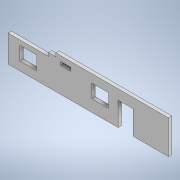
# Autodesk Inventor part: westSideofHouseFacingGarage
Saved by Autodesk Inventor 2020.1 (Build 241239000, 239)
## iProperties
Created: 2019-08-10
Part Number: westSideofHouseFacingGarage
Material: Generic
Document SubType Name: Modeling
Designer: steele
Density: 1 g/cm^3
Appearance: Default
Author: steele
Autodesk Inventor part; units mm, degrees
ref_plane "YZ Plane" through (0, 0, 0) normal (1, 0, 0) x (0, 1, 0)
ref_plane "XZ Plane" through (0, 0, 0) normal (0, 1, 0) x (-1, 0, 0)
ref_plane "XY Plane" through (0, 0, 0) normal (0, 0, 1) x (1, 0, 0)
sketch "Sketch1" plane through (0, 0, 0) normal (0, 0, 1) x (1, 0, 0)
  line L0 (0, 0) -> (3657.6, 0)
  line L1 (3657.6, 0) -> (3657.6, 2438.4)
  line L2 (3657.6, 2438.4) -> (0, 2438.4)
  line L3 (0, 2438.4) -> (0, 0)
  line L4 (3657.6, 0) -> (4318, 0)
  line L5 (4318, 2743.2) -> (3657.6, 2743.2)
  line L6 (3657.6, 2743.2) -> (3657.6, 0)
  line L7 (4318, 0) -> (9956.8, 0)
  line L8 (9956.8, 0) -> (9956.8, 2159)
  line L9 (9956.8, 3048) -> (4318, 3048)
  line L10 (4318, 3048) -> (4318, 0)
  line L11 (9956.8, 0) -> (11328.4, 0)
  line L12 (11328.4, 0) -> (11328.4, 2159)
  line L13 (11328.4, 2159) -> (9956.8, 2159)
  line L14 (9956.8, 2159) -> (9956.8, 0)
  line L15 (9956.8, 0) -> (14528.8, 0)
  line L16 (14528.8, 0) -> (14528.8, 3048)
  line L17 (14528.8, 3048) -> (9956.8, 3048)
  line L18 (9956.8, 3048) -> (9956.8, 0)
  line L19 (4775.2, 2286) -> (5689.6, 2286)
  line L20 (5689.6, 2286) -> (5689.6, 2590.8)
  line L21 (5689.6, 2590.8) -> (4775.2, 2590.8)
  line L22 (4775.2, 2590.8) -> (4775.2, 2286)
  line L23 (4775.2, 2286) -> (5689.6, 2590.8) construction
  line L24 (5689.6, 2286) -> (4775.2, 2590.8) construction
  line L25 (7567.3793, 1088.0908) -> (9091.3793, 1088.0908)
  line L26 (9091.3793, 1088.0908) -> (9091.3793, 2307.2908)
  line L27 (9091.3793, 2307.2908) -> (7567.3793, 2307.2908)
  line L28 (7567.3793, 2307.2908) -> (7567.3793, 1088.0908)
  line L29 (7567.3793, 1088.0908) -> (9091.3793, 2307.2908) construction
  line L30 (9091.3793, 1088.0908) -> (7567.3793, 2307.2908) construction
  line L31 (1066.8, 792.7558) -> (2590.8, 792.7558)
  line L32 (2590.8, 792.7558) -> (2590.8, 2011.9558)
  line L33 (2590.8, 2011.9558) -> (1066.8, 2011.9558)
  line L34 (1066.8, 2011.9558) -> (1066.8, 792.7558)
  line L35 (1066.8, 792.7558) -> (2590.8, 2011.9558) construction
  line L36 (2590.8, 792.7558) -> (1066.8, 2011.9558) construction
  line L37 (4318, 0) -> (4318, 2159)
  line L38 (4318, 2286) -> (4318, 2743.2)
  point P0 (5232.4, 2438.4)
  point P1 (8329.3793, 1697.6908)
  point P2 (1828.8, 1402.3558)
  dimension "d0" = 3657.6
  dimension "d1" = 2438.4
  dimension "d2" = 660.4
  dimension "d3" = 2743.2
  dimension "d4" = 5638.8
  dimension "d5" = 3048
  dimension "d6" = 1371.6
  dimension "d7" = 2159
  dimension "d8" = 4572
  dimension "d9" = 3048
  dimension "d10" = 304.8
  dimension "d11" = 914.4
  dimension "d14" = 1524
  dimension "d15" = 1219.2
  dimension "d16" = 1524
  dimension "d17" = 1219.2
  dimension "d18" = 1828.8
  dimension "d19" = 3200.4
  dimension "d22" = 14528.8
  constraints: 78 end point, 17 parallel, 9 perpendicular, 8 horizontal, 6 midpoint, 2 point on line
  measures "d0" distance of L2.end L1.end
  measures "d1" distance of L1.end L0.end
  measures "d2" distance of L5.end L5.start
  measures "d3" distance of L5.start L4.end
  measures "d4" distance of L9.end L9.start
  measures "d5" distance of L9.start L7.end
  measures "d6" distance of L8.end L12.end
  measures "d7" distance of L12.end L11.end
  measures "d8" distance of L17.end L16.end
  measures "d9" distance of L16.end L15.end
  measures "d10" distance of L19.end L20.end
  measures "d11" distance of L19.start L19.end
  measures "d14" distance of L25.start L25.end
  measures "d15" distance of L26.end L25.end
  measures "d16" distance of L31.start L31.end
  measures "d17" distance of L32.end L31.end
  measures "d18" distance from line of point (1828.8, 1402.356) L3
  measures "d19" distance between parallel lines of L16 L12
  measures "d22" distance of L15.end L0.start
extrude "Extrusion1" add sketch "Sketch1" against normal blind 304.8 contours L3 L2 L1 L0 | L1 L6 L5 L10 L4 | L10 L9 L18 L8 L7 | L18 L17 L16 L15 L12 L13
body "Solid1"
